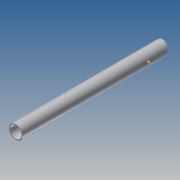
# Autodesk Inventor part: 2p5vss
Saved by Autodesk Inventor 2014 SP1 (Build 180222100, 222)
## iProperties
Company: HERA Project
Created: 2013-06-11
Part Number: 2p5vss
Material: PVC-Piping
Document SubType Name: Modeling
Designer: David DeBoer
Density: 1.4 g/cm^3
Description: support vertical spar
Mass: 468.384 g
Surface Area: 1724.47 cm^2
Volume: 334.56 cm^3
Appearance: Smooth - White
Author: David DeBoer
Title: Hub-supporthold
Autodesk Inventor part; units mm, degrees
ref_plane "YZ Plane" through (0, 0, 0) normal (1, 0, 0) x (0, 1, 0)
ref_plane "XZ Plane" through (0, 0, 0) normal (0, 1, 0) x (-1, 0, 0)
ref_plane "XY Plane" through (0, 0, 0) normal (0, 0, 1) x (1, 0, 0)
sketch "Sketch1" plane through (0, 0, 0) normal (0, 0, 1) x (1, 0, 0)
  circle A0 centre (0, 0) radius 30.1625
  circle A1 centre (0, 0) radius 26.2509
  dimension "d0" = 60.325
  dimension "d2" = 3.9116
  constraints: 2 centre point, 1 coincident
  measures "d0" diameter of A0
  measures "d2" radial gap between concentric circles of A1 A0
extrude "Extrusion1" add sketch "Sketch1" along normal blind 691.388
sketch "Sketch15" plane through (0, 0, 691.388) normal (0, 0, 1) x (1, 0, 0)
  circle A0 centre (0, 0) radius 26.2509 projected
  circle A1 centre (0, 0) radius 30.1625 projected
  point P0 (30.1625, 0)
  constraints: 1 horizontal alignment, 1 other
ref_plane "Work Plane6" through (30.1625, 0, 691.388) normal (1, 0, 0) x (0, 1, 0)
sketch "Sketch16" plane through (30.1625, 0, 691.388) normal (1, 0, 0) x (0, 1, 0)
  line L0 (0, -691.388) -> (-41.9813, -691.388)
  line L1 (-41.9813, -691.388) -> (-41.9813, -627.8327)
  line L2 (-41.9813, -627.8327) -> (53.6182, -662.2317)
  line L3 (53.6182, -662.2317) -> (53.6182, -691.388)
  line L4 (53.6182, -691.388) -> (0, -691.388)
  dimension "d51" = 101.6
  dimension "d52" = 70.21
  constraints: 10 end point, 1 collinear, 1 horizontal, 1 parallel, 1 perpendicular
  measures "d51" distance of L1.end L2.end
  measures "d52" angle of L1 L2
extrude "Extrusion9" cut sketch "Sketch16" against normal blind 101.6
sketch "Sketch17" plane through (30.1625, 0, 691.388) normal (1, 0, 0) x (0, 1, 0)
  line L0 (-26.6972, -579.592) -> (25.3008, -579.592) construction
  point P0 (0, -691.388)
  constraints: 2 end point, 1 horizontal
sketch "Sketch18" plane through (30.1625, 0, 691.388) normal (1, 0, 0) x (0, 1, 0)
  circle A0 centre (-6.35, -589.788) radius 2.1594
  circle A1 centre (6.35, -558.038) radius 3.1512
  point P0 (0, -691.388)
  dimension "d55" = 6.35
  dimension "d56" = 12.7
  dimension "d57" = 31.75
  dimension "d65" = 101.6
  constraints: 2 centre point
  measures "d55" horizontal distance of A0.centre point (0, -691.388)
  measures "d56" horizontal distance of A1.centre A0.centre
  measures "d57" vertical distance of A1.centre A0.centre
  measures "d65" vertical distance of point (0, -691.388) A0.centre
hole "Hole1" at (30.1625, 6.35, 133.35) at (30.1625, -6.35, 101.6) direction (-1, 0, 0) diameter 1.5875 end through all
body "Solid1"
